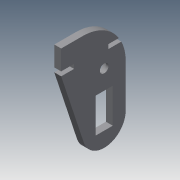
# Autodesk Inventor part: sablona-packa-strana1
Saved by Autodesk Inventor 2013 (Build 170138000, 138)
## iProperties
Created: 2013-05-25
Part Number: sablona-packa-strana1
Material: Generic
Document SubType Name: Modeling
Designer: idle-rug
Density: 1 g/cm^3
Author: idle-rug
Autodesk Inventor part; units mm, degrees
ref_plane "YZ Plane" through (0, 0, 0) normal (1, 0, 0) x (0, 1, 0)
ref_plane "XZ Plane" through (0, 0, 0) normal (0, 1, 0) x (-1, 0, 0)
ref_plane "XY Plane" through (0, 0, 0) normal (0, 0, 1) x (1, 0, 0)
sketch "Sketch1" plane through (0, 0, 0) normal (1, 0, 0) x (0, 1, 0)
  circle A0 centre (0, 0) radius 16.575
  line L0 (0, 16.575) -> (0, -49.725)
  line L1 (0, -33.15) -> (0, -15.05)
  line L2 (0, -15.05) -> (0, -70.05)
  line L3 (10, -70.05) -> (-10, -70.05)
  line L4 (-10, -70.05) -> (-10, -15.05)
  line L5 (-10, -15.05) -> (10, -15.05)
  line L6 (10, -15.05) -> (10, -70.05)
  line L7 (10, -70.05) -> (-10, -15.05) construction
  line L8 (-10, -70.05) -> (10, -15.05) construction
  line L9 (10, -62.65) -> (-10, -62.65)
  line L10 (-10, -62.65) -> (-10, -22.45)
  line L11 (-10, -22.45) -> (10, -22.45)
  line L12 (10, -22.45) -> (10, -62.65)
  line L13 (10, -62.65) -> (-10, -22.45) construction
  line L14 (-10, -62.65) -> (10, -22.45) construction
  line L15 (-4.95, -27.2) -> (-4.95, -17.7)
  line L16 (-4.95, -17.7) -> (4.95, -17.7)
  line L17 (4.95, -27.2) -> (-4.95, -17.7) construction
  line L18 (-4.95, -27.2) -> (4.95, -17.7) construction
  line L19 (4.95, -67.4) -> (-4.95, -67.4)
  line L20 (-4.95, -67.4) -> (-4.95, -57.9)
  line L21 (-4.95, -57.9) -> (4.95, -57.9)
  line L22 (4.95, -67.4) -> (-4.95, -57.9) construction
  line L23 (-4.95, -67.4) -> (4.95, -57.9) construction
  circle A1 centre (4.95, -17.7) radius 1.5
  circle A2 centre (-4.95, -17.7) radius 1.5
  circle A3 centre (4.95, -67.4) radius 1.5
  circle A4 centre (-4.95, -67.4) radius 1.5
  circle A5 centre (0, -33.15) radius 6.8
  line L24 (0, -80) -> (0, -55)
  arc A6 (-25, -55) -> (25, -55) centre (0, -55) ccw
  line L25 (0, 0) -> (0, 45)
  line L26 (25, 45) -> (-25, 45)
  line L27 (25, 45) -> (25, -55)
  line L28 (-25, 45) -> (-25, -55)
  circle A7 centre (0, 0) radius 7.5
  point P0 (0, -42.55)
  point P1 (0, -42.55)
  point P2 (0, -22.45)
  point P3 (0, -62.65)
  dimension "d0" = 33.15
  dimension "d2" = 66.3
  dimension "d4" = 18.1
  dimension "d5" = 55
  dimension "d6" = 20
  dimension "d7" = 55
  dimension "d8" = 40.2
  dimension "d9" = 9.9
  dimension "d10" = 9.5
  dimension "d11" = 9.9
  dimension "d12" = 9.5
  dimension "d13" = 3
  dimension "d14" = 3
  dimension "d15" = 3
  dimension "d16" = 3
  dimension "d17" = 13.6
  dimension "d20" = 25
  dimension "d21" = 45
  dimension "d22" = 15
  constraints: 58 end point, 12 midpoint, 7 centre point, 7 coincident, 6 parallel, 6 point on line, 4 perpendicular, 3 horizontal, 2 point on circle, 2 tangent, 1 vertical, 1 vertical alignment, 2 other
  measures "d2" distance of L0.start L0.end
  measures "d4" distance of L1.start L1.end
  measures "d5" distance of L1.end L2.end
  measures "d6" distance of L4.end L5.end
  measures "d7" distance of L3.end L4.end
  measures "d8" distance of L9.end L10.end
  measures "d9" distance of L15.end L16.end
  measures "d10" distance of L15.start L15.end
  measures "d11" distance of L20.end L21.end
  measures "d12" distance of L19.end L20.end
  measures "d13" diameter of A1
  measures "d14" diameter of A2
  measures "d15" diameter of A3
  measures "d16" diameter of A4
  measures "d17" diameter of A5
  measures "d20" distance of L24.start L24.end
  measures "d21" distance of L25.start L25.end
  measures "d22" diameter of A7
extrude "Extrusion1" add sketch "Sketch1" along normal blind 5 contours A0 L5 L0 A7 | A0 L25 L26 L27 A6 L24 L3 L6 L5 | L0 A7 L5 A0 | A0 L5 L4 L3 L24 A6 L28 L26 L25 | L5 L6 L11 L0 A0 | A0 L0 L5 | L5 L0 A0 | A0 L0 L16 A2 L15 L11 L4 L5 | L0 L11 L15 A2 L16 | L6 L9 L2 L0 A5 L11 | L11 L0 A5 L2 L21 L20 L9 L4 | L6 L3 L2 L9 | L9 L20 A4 L19 L2 L3 L4 | L9 L20 L21 L2 | L2 L19 A4 L20 L9
sketch "Sketch2" plane through (5, 0, 0) normal (1, 0, 0) x (0, 0, -1)
  line L0 (-45, -25) -> (55, -25) projected
  circle A0 centre (33.15, 0) radius 6.8 projected
  line L1 (33.15, 0) -> (15.05, 0)
  line L2 (15.05, 0) -> (70.05, 0)
  line L3 (62.65, 10) -> (22.45, 10)
  line L4 (22.45, 10) -> (22.45, -10)
  line L5 (22.45, -10) -> (62.65, -10)
  line L6 (62.65, -10) -> (62.65, 10)
  line L7 (62.65, 10) -> (22.45, -10) construction
  line L8 (22.45, 10) -> (62.65, -10) construction
  point P0 (42.55, 0)
  dimension "d25" = 18.1
  dimension "d26" = 55
  dimension "d27" = 40.2
  dimension "d28" = 20
  constraints: 16 end point, 3 midpoint, 3 parallel, 1 collinear, 1 horizontal, 1 perpendicular
  measures "d25" distance of L1.start L1.end
  measures "d26" distance of L1.end L2.end
  measures "d27" distance of L5.end L4.end
  measures "d28" distance of L4.end L3.end
extrude "Extrusion2" cut sketch "Sketch2" against normal blind 5 contours L2 L6 L5 L4 L1 A0 | A0 L1 L4 L3 L6 L2
sketch "Sketch3" plane through (5, 0, 0) normal (1, 0, 0) x (0, 0, -1)
  circle A0 centre (17.7, 4.95) radius 1.5 projected
  circle A1 centre (17.7, -4.95) radius 1.5 projected
  circle A2 centre (67.4, 4.95) radius 1.5 projected
  circle A3 centre (67.4, -4.95) radius 1.5 projected
extrude "Extrusion3" add sketch "Sketch3" against normal blind 5
sketch "Sketch4" plane through (5, 0, 0) normal (1, 0, 0) x (0, 0, -1)
  line L0 (55, 25) -> (-45, 25) projected
  line L1 (-45, 25) -> (-45, -25) projected
  line L2 (-45, -25) -> (55, -25) projected
  line L3 (-45, 25) -> (-35, 25)
  line L4 (-35, 25) -> (-35, -25)
  line L5 (-35, -25) -> (-45, -25)
  line L6 (-45, -25) -> (-45, 25)
  dimension "d33" = 10
  constraints: 8 end point, 2 collinear, 2 point on line, 1 perpendicular
  measures "d33" distance of L0.end L3.end
extrude "Extrusion4" add sketch "Sketch4" along normal blind 32.9
sketch "Sketch5" plane through (0, -25, -55) normal (0, -1, 0) x (1, 0, 0)
  line L0 (5, 90) -> (37.9, 90)
  line L1 (37.9, 90) -> (37.9, 100)
  line L2 (37.9, 100) -> (5, 100)
  line L3 (5, 100) -> (5, 90)
  point P0 (0, 55)
  constraints: 8 end point, 2 parallel, 1 horizontal, 1 perpendicular
extrude "Extrusion5" add sketch "Sketch5" along normal blind 25
sketch "Sketch6" plane through (0, 0, 0) normal (-1, 0, 0) x (0, 0, 1)
  arc A0 (-55, 25) -> (-55, -25) centre (-55, 0) ccw projected
  line L0 (45, -25) -> (-55, -25) projected
  line L1 (-55, 25) -> (45, 25) projected
  line L2 (45, -25) -> (45, -50)
  line L3 (45, -50) -> (35, -50)
  line L4 (35, -50) -> (-61.4711, -24.148)
  line L5 (-55, -25) -> (45, -25)
  arc A1 (-61.4711, -24.148) -> (-55, -25) centre (-55, 0) ccw
  dimension "d38" = 25
  dimension "d39" = 10
  constraints: 8 end point, 3 point on circle, 3 tangent, 2 perpendicular, 1 centre point, 1 collinear, 1 concentric
  measures "d38" distance of L0.start L2.end
  measures "d39" distance of L2.end L3.end
extrude "Extrusion6" add sketch "Sketch6" against normal blind 5
sketch "Sketch7" plane through (0, 25, 45) normal (0, 0, 1) x (1, 0, 0)
  line L0 (37.9, -75) -> (0, -75) projected
  line L1 (0, 0) -> (37.9, 0) projected
  line L2 (18.95, -75) -> (18.95, -62.5)
  circle A0 centre (18.95, -62.5) radius 7.5
  point P0 (0, -25)
  dimension "d42" = 12.5
  dimension "d43" = 15
  constraints: 2 end point, 1 centre point, 1 coincident, 1 midpoint, 1 perpendicular
  measures "d42" distance of L2.start L2.end
  measures "d43" diameter of A0
extrude "Extrusion7" cut sketch "Sketch7" against normal blind 10
sketch "Sketch8" plane through (5, 0, 0) normal (1, 0, 0) x (0, 0, -1)
  line L0 (-35, 25) -> (-35, -50) projected
  line L1 (55, 25) -> (-35, 25) projected
  line L2 (-35, -50) -> (-35, 25)
  line L3 (-35, -50) -> (-17, -50)
  line L4 (-17, -50) -> (-17, 25)
  line L5 (-17, -50) -> (61.4711, -24.148)
  line L6 (-17, -50) -> (-22, -50)
  line L7 (-22, -50) -> (-22, 25)
  line L8 (-17, 25) -> (-22, 25)
  dimension "d46" = 18
  dimension "d47" = 5
  constraints: 14 end point, 4 perpendicular, 3 point on line, 1 collinear
  measures "d46" distance of L0.end L3.end
  measures "d47" distance of L3.end L6.end
extrude "Extrusion8" add sketch "Sketch8" along normal blind 32.9 contours L1 L4 L3 L7
sketch "Sketch9" plane through (0, 0, 0) normal (-1, 0, 0) x (0, 0, 1)
  line L0 (-61.4711, -24.148) -> (35, -50) projected
  arc A0 (-55, 25) -> (-61.4711, -24.148) centre (-55, 0) ccw projected
  line L1 (17, -50) -> (-61.4711, -24.148)
  line L2 (-61.4711, -24.148) -> (35, -50)
  line L3 (35, -50) -> (17, -50)
  line L4 (35, -50) -> (17, -50)
  line L5 (17, -50) -> (-61.4711, -24.148)
  line L6 (-61.4711, -24.148) -> (35, -50)
  point P0 (45, -50)
  dimension "d50" = 28
  constraints: 12 end point, 4 collinear, 2 tangent, 1 point on circle
  measures "d50" distance of point (45, -50) L1.start
extrude "Extrusion9" add sketch "Sketch9" against normal blind 5
sketch "Sketch11" plane through (0, 25, 45) normal (0, 0, 1) x (1, 0, 0)
  circle A0 centre (18.95, -62.5) radius 7.5 projected
  point P0 (0, -25)
extrude "Extrusion10" add sketch "Sketch11" against normal blind 10
sketch "Sketch12" plane through (0, 25, 45) normal (0, 0, 1) x (1, 0, 0)
  line L0 (37.9, -75) -> (0, -75) projected
  line L1 (0, -75) -> (5, -75)
  line L2 (37.9, -75) -> (5, -75)
  line L3 (21.45, -75) -> (21.45, -62.5)
  circle A0 centre (21.45, -62.5) radius 6.8
  point P0 (0, -25)
  dimension "d55" = 5
  dimension "d56" = 12.5
  dimension "d57" = 13.6
  constraints: 6 end point, 1 centre point, 1 coincident, 1 collinear, 1 midpoint, 1 perpendicular, 1 point on line
  measures "d55" distance of L0.end L1.end
  measures "d56" distance of L3.start L3.end
  measures "d57" diameter of A0
extrude "Extrusion11" cut sketch "Sketch12" against normal blind 10
sketch "Sketch13" plane through (37.9, 25, 17) normal (0, 0, -1) x (-1, 0, 0)
  line L0 (32.9, -75) -> (0, -75) projected
  line L1 (16.45, -75) -> (16.45, -62.5)
  circle A0 centre (16.45, -62.5) radius 6.2
  line L2 (16.45, -62.5) -> (16.45, -50.3)
  circle A1 centre (16.45, -56.4) radius 3.1
  point P0 (37.9, -25)
  dimension "d60" = 12.5
  dimension "d61" = 12.4
  dimension "d62" = 12.2
  dimension "d63" = 6.2
  constraints: 4 end point, 2 centre point, 2 midpoint, 1 coincident, 1 collinear, 1 perpendicular
  measures "d60" distance of L1.start L1.end
  measures "d61" diameter of A0
  measures "d62" distance of L2.start L2.end
  measures "d63" diameter of A1
extrude "Extrusion12" cut sketch "Sketch13" against normal blind 5
sketch "Sketch15" plane through (37.9, 25, 17) normal (0, 0, -1) x (-1, 0, 0)
  arc A0 (13.4271, -57.0869) -> (19.4729, -57.0869) centre (16.45, -62.5) ccw projected
  line L0 (32.9, -75) -> (0, -75) projected
  line L1 (16.45, -62.5) -> (16.45, -73.1)
  circle A1 centre (16.45, -73.1) radius 1
  line L2 (16.45, -62.5) -> (16.45, -41.1)
  circle A2 centre (16.45, -41.1) radius 1
  point P0 (37.9, -25)
  dimension "d66" = 10.6
  dimension "d67" = 2
  dimension "d68" = 21.4
  dimension "d69" = 2
  constraints: 4 end point, 2 centre point, 2 coincident, 1 collinear, 1 perpendicular
  measures "d66" distance of L1.start L1.end
  measures "d67" diameter of A1
  measures "d68" distance of L1.start L2.end
  measures "d69" diameter of A2
extrude "Extrusion13" cut sketch "Sketch15" against normal blind 5
sketch "Sketch16" plane through (37.9, 25, 17) normal (0, 0, -1) x (-1, 0, 0)
  circle A0 centre (16.45, -73.1) radius 1 projected
  circle A1 centre (16.45, -41.1) radius 1 projected
  line L0 (32.9, -75) -> (0, -75) projected
  line L1 (16.45, -41.1) -> (16.45, -43.15)
  line L2 (16.45, -73.1) -> (16.45, -71.05)
  point P0 (37.9, -25)
  dimension "d72" = 2.05
  dimension "d73" = 2.05
  constraints: 4 end point, 1 collinear, 1 perpendicular
  measures "d72" distance of L1.start L1.end
  measures "d73" distance of L2.start L2.end
extrude "Extrusion14" add sketch "Sketch16" against normal blind 5
sketch "Sketch17" plane through (37.9, 25, 17) normal (0, 0, -1) x (-1, 0, 0)
  arc A0 (13.4271, -57.0869) -> (19.4729, -57.0869) centre (16.45, -62.5) ccw projected
  line L0 (32.9, -75) -> (0, -75) projected
  line L1 (16.45, -62.5) -> (16.45, -41.1)
  line L2 (16.45, -41.1) -> (16.45, -43.15)
  circle A1 centre (16.45, -43.15) radius 1
  line L3 (16.45, -62.5) -> (16.45, -73.1)
  line L4 (16.45, -73.1) -> (16.45, -71.05)
  circle A2 centre (16.45, -71.05) radius 1
  point P0 (37.9, -25)
  dimension "d76" = 21.4
  dimension "d77" = 2.05
  dimension "d78" = 2
  dimension "d79" = 10.6
  dimension "d80" = 2.05
  dimension "d81" = 2
  constraints: 8 end point, 2 centre point, 2 coincident, 2 point on line, 1 collinear, 1 perpendicular
  measures "d76" distance of L1.start L1.end
  measures "d77" distance of L1.end L2.end
  measures "d78" diameter of A1
  measures "d79" distance of L1.start L3.end
  measures "d80" distance of L3.end L4.end
  measures "d81" diameter of A2
extrude "Extrusion15" cut sketch "Sketch17" against normal blind 5
sketch "Sketch18" plane through (0, 0, 0) normal (-1, 0, 0) x (0, 0, 1)
  line L0 (45, 25) -> (45, -50) projected
  line L1 (-55, 25) -> (45, 25) projected
  line L2 (45, 25) -> (45, -20)
  line L3 (45, 25) -> (0, 25)
  line L4 (0, 25) -> (-5, 25)
  line L5 (45, -20) -> (45, -25)
  arc A0 (45, -25) -> (-5, 25) centre (-5, -25) ccw
  dimension "d84" = 45
  dimension "d86" = 5
  dimension "d87" = 5
  constraints: 8 end point, 3 point on line, 2 point on circle, 2 tangent, 1 centre point, 1 midpoint
  measures "d84" distance of L0.start L2.end
  measures "d86" distance of L3.end L4.end
  measures "d87" distance of L2.end L5.end
extrude "Extrusion16" cut sketch "Sketch18" against normal blind 39
sketch "Sketch19" plane through (37.9, -50, 17) normal (0, 0, -1) x (-1, 0, 0)
  line L0 (32.9, 0) -> (32.9, 69.8999) projected
  arc A0 (13.4271, 17.9131) -> (19.4729, 17.9131) centre (16.45, 12.5) ccw projected
  arc A1 (19.4729, 17.9131) -> (13.4271, 17.9131) centre (16.45, 18.6) ccw projected
  line L1 (0, 25) -> (0, 0) projected
  line L2 (0, 6.3) -> (32.9, 6.3)
  line L3 (0, 6.3) -> (0, 28.3)
  line L4 (0, 55) -> (0, 25) projected
  line L5 (0, 28.3) -> (32.9, 28.3)
  line L6 (32.9, 28.3) -> (32.9, 6.3)
  point P0 (37.9, 50)
  dimension "d90" = 22
  constraints: 8 end point, 4 point on line, 2 perpendicular
  measures "d90" distance of L2.start L3.end
extrude "Extrusion17" cut sketch "Sketch19" against normal blind 5
sketch "Sketch21" plane through (5, 0, 0) normal (1, 0, 0) x (0, 0, -1)
  line L0 (22.45, -10) -> (22.45, 10) projected
  line L1 (22.45, 10) -> (62.65, 10) projected
  line L2 (62.65, 10) -> (62.65, -10) projected
  line L3 (62.65, -10) -> (22.45, -10) projected
  circle A0 centre (0, 0) radius 7.5 projected
  arc A1 (-22, 17.0833) -> (-35, 5) centre (5, -25) ccw projected
  line L4 (-35, 5) -> (-35, -50) projected
  line L5 (-35, -50) -> (-22, -50) projected
  line L6 (-22, -43.7) -> (-22, -50) projected
  line L7 (-17, -43.7) -> (-22, -43.7) projected
  line L8 (-17, -50) -> (-17, -43.7) projected
  line L9 (-17, -50) -> (61.4711, -24.148) projected
  arc A2 (61.4711, -24.148) -> (55, 25) centre (55, 0) ccw projected
  line L10 (55, 25) -> (5, 25) projected
  arc A3 (5, 25) -> (-17, 19.8999) centre (5, -25) ccw projected
  line L11 (-17, -21.7) -> (-17, 19.8999) projected
  line L12 (-17, -21.7) -> (-22, -21.7) projected
  line L13 (-22, 17.0833) -> (-22, -21.7) projected
extrude "Extrusion18" add sketch "Sketch21" along normal blind 3
sketch "Sketch22" plane through (0, -50, 45) normal (0, 0, 1) x (1, 0, 0)
  circle A0 centre (21.45, 12.5) radius 6.8 projected
  circle A1 centre (21.45, 12.5) radius 5
  point P0 (0, 50)
  dimension "d95" = 10
  constraints: 1 centre point, 1 coincident
  measures "d95" diameter of A1
extrude "Extrusion19" add sketch "Sketch22" against normal blind 2
sketch "Sketch23" plane through (37.9, -50, 35) normal (0, 0, -1) x (-1, 0, 0)
  circle A0 centre (16.45, 12.5) radius 6.8 projected
  line L0 (29.9, 0) -> (29.9, 55) projected
  line L1 (29.9, 55) -> (0, 55) projected
  line L2 (0, 55) -> (0, 0) projected
  line L3 (29.9, 0) -> (0, 0) projected
  point P0 (37.9, 50)
extrude "Extrusion20" add sketch "Sketch23" along normal blind 2
sketch "Sketch24" plane through (37.9, -21.7, 17) normal (0, -1, 0) x (1, 0, 0)
  line L0 (-29.9, 5) -> (0, 5) projected
  line L1 (0, 0) -> (-10.25, 0)
  line L2 (-10.25, 0) -> (-10.25, 5)
  line L3 (-10.25, 5) -> (0, 5)
  line L4 (0, 5) -> (0, 0)
  line L5 (-29.9, 0) -> (-22.65, 0)
  line L6 (-22.65, 0) -> (-22.65, 5)
  line L7 (-22.65, 5) -> (-29.9, 5)
  line L8 (-29.9, 5) -> (-29.9, 0)
  point P0 (-37.9, -17)
  dimension "d100" = 10.25
  dimension "d101" = 7.25
  constraints: 16 end point, 4 parallel, 2 horizontal, 2 perpendicular, 2 point on line
  measures "d100" distance of L2.end L3.end
  measures "d101" distance of L7.end L6.end
extrude "Extrusion21" add sketch "Sketch24" along normal blind 22
sketch "Sketch25" plane through (37.9, -50, 33) normal (0, 0, -1) x (-1, 0, 0)
  circle A0 centre (16.45, 12.5) radius 6.8 projected
  circle A1 centre (16.45, 12.5) radius 5
  point P0 (37.9, 50)
  dimension "d104" = 10
  constraints: 1 centre point, 1 coincident
  measures "d104" diameter of A1
extrude "Extrusion22" add sketch "Sketch25" against normal blind 2
sketch "Sketch26" plane through (8, 0, 0) normal (1, 0, 0) x (0, 0, -1)
  circle A0 centre (0, 0) radius 7.5 projected
  circle A1 centre (0, 0) radius 5
  dimension "d107" = 10
  constraints: 1 centre point, 1 coincident
  measures "d107" diameter of A1
extrude "Extrusion23" add sketch "Sketch26" against normal blind 3
sketch "Sketch28" plane through (37.9, -50, 17) normal (0, 0, -1) x (-1, 0, 0)
  line L0 (10.25, 28.3) -> (10.25, 6.3) projected
  line L1 (22.65, 28.3) -> (22.65, 6.3) projected
  arc A0 (22.65, 6.3) -> (22.65, 28.3) centre (13.9897, 17.3) ccw
  arc A1 (10.25, 28.3) -> (10.25, 6.3) centre (18.9103, 17.3) ccw
  point P0 (37.9, 50)
  dimension "d111" = 14
  dimension "d112" = 14
  constraints: 4 point on circle, 2 centre point
  measures "d111" radius of A0
  measures "d112" radius of A1
extrude "Extrusion24" cut sketch "Sketch28" against normal blind 5
sketch "Sketch29" plane through (37.9, 0, 0) normal (1, 0, 0) x (0, 0, -1)
  line L0 (-22, 17.0833) -> (-22, -50) projected
  line L1 (-22, -50) -> (-17, -50) projected
  line L2 (-17, -50) -> (-17, 19.8999) projected
  arc A0 (-17, 19.8999) -> (-22, 17.0833) centre (5, -25) ccw projected
  line L3 (-22, -50) -> (-22, -35)
  line L4 (-22, -35) -> (-17, -35)
  line L5 (-22, -50) -> (-17, -50)
  line L6 (-17, -50) -> (-17, -35)
  line L7 (-17, 19.8999) -> (-17, 4.8999)
  line L8 (-17, 4.8999) -> (-22, 4.8999)
  line L9 (-22, 4.8999) -> (-22, 17.0833)
  point P0 (0, 0)
  dimension "d115" = 15
  dimension "d116" = 15
  constraints: 15 end point, 4 point on line, 2 collinear, 2 perpendicular
  measures "d115" distance of L0.end L3.end
  measures "d116" distance of L2.end L7.end
extrude "Extrusion25" cut sketch "Sketch29" against normal blind 37.9 contours A0 L2 L8 L0 | L4 L2 L1 L0
sketch "Sketch30" plane through (37.9, 0, 0) normal (1, 0, 0) x (0, 0, -1)
  line L0 (-17, 4.8999) -> (-22, 4.8999) projected
  line L1 (-22, 4.8999) -> (-22, -35) projected
  line L2 (-22, -35) -> (-17, -35) projected
  line L3 (-17, -35) -> (-17, 4.8999) projected
  point P0 (0, 0)
extrude "Extrusion26" cut sketch "Sketch30" against normal blind 29.9
sketch "Sketch32" plane through (8, 0, 0) normal (1, 0, 0) x (0, 0, -1)
  arc A0 (-22, 17.0833) -> (-35, 5) centre (5, -25) ccw projected
  line L0 (-35, 5) -> (-33, 5) projected
  line L1 (-33, 5) -> (-33, -50) projected
  line L2 (-22, 4.8999) -> (-17, 4.8999) projected
  line L3 (-33, 5) -> (-33, 7.4962)
  line L4 (-33, 7.4962) -> (-33, -50)
  line L5 (-33, -50) -> (-45, -50)
  line L6 (-45, -50) -> (-33, -50) projected
  constraints: 6 end point, 2 collinear, 1 perpendicular, 1 point on circle
extrude "Extrusion27" add sketch "Sketch32" along normal blind 29.9
sketch "Sketch33" plane through (37.9, 0, 0) normal (1, 0, 0) x (0, 0, -1)
  arc A0 (-33, 7.4962) -> (-45, -25) centre (5, -25) ccw projected
  line L0 (-45, -25) -> (-45, -50) projected
  line L1 (-45, -50) -> (-33, -50) projected
  line L2 (-33, -50) -> (-33, 7.4962) projected
  point P0 (0, 0)
extrude "Extrusion28" cut sketch "Sketch33" against normal blind 29.9
body "Solid1"
